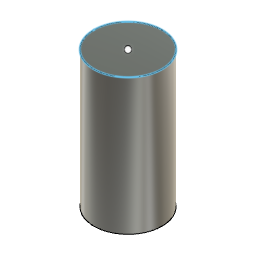
Pilon 2 (Autodesk Fusion 360 design; units mm, degrees)
Autodesk Fusion 360 part; units mm, degrees
sketch "sketch 309" plane through (0, 0, 15) normal (0, 0, 1) x (-1, 0, 0)
  circle A0 centre (-87.5, -105) radius 2.5
  circle A1 centre (-87.5, -105) radius 2.5
extrude "Extrude1" add sketch "sketch 309" along normal blind -10 and the other way blind -5
extrude "Extrude2" cut 1 faces at (85.7397, 105.1944, 20) along direction (0, 0, -1) blind 5
